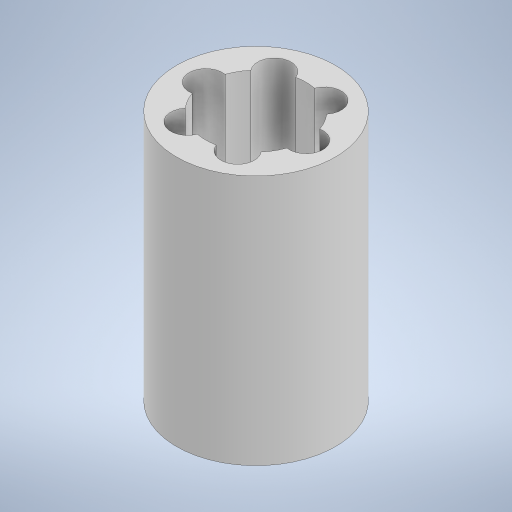
# Autodesk Inventor part: Bearing
Saved by Autodesk Inventor 2023 (Build 270158000, 158)
## iProperties
Created: 2023-04-11
Part Number: Bearing
Material: Generic
Document SubType Name: Modeling
Designer: Nathann
Density: 1 g/cm^3
Appearance: Default
Author: Nathann
Autodesk Inventor part; units mm, degrees
ref_plane "YZ Plane" through (0, 0, 0) normal (1, 0, 0) x (0, 1, 0)
ref_plane "XZ Plane" through (0, 0, 0) normal (0, 1, 0) x (-1, 0, 0)
ref_plane "XY Plane" through (0, 0, 0) normal (0, 0, 1) x (1, 0, 0)
sketch "Sketch1" plane through (0, 0, 0) normal (0, 1, 0) x (-1, 0, 0)
  circle A0 centre (0, 0) radius 6
  circle A1 centre (0, 0) radius 9.5
  circle A2 centre (6, 0) radius 2
  circle A3 centre (3, 5.1962) radius 2
  circle A4 centre (-3, 5.1962) radius 2
  circle A5 centre (-6, 0) radius 2
  circle A6 centre (-3, -5.1962) radius 2
  circle A7 centre (3, -5.1962) radius 2
  point P0 (5.6667, -1.972)
  point P1 (5.6667, 1.972)
  point P2 (4.5412, -3.9215)
  point P3 (1.1255, -5.8935)
  point P4 (-1.1255, -5.8935)
  point P5 (-4.5412, -3.9215)
  point P6 (-5.6667, -1.972)
  point P7 (-5.6667, 1.972)
  point P8 (-4.5412, 3.9215)
  point P9 (-1.1255, 5.8935)
  point P10 (1.1255, 5.8935)
  point P11 (4.5412, 3.9215)
  dimension "d1" = 12
  dimension "d0" = 19
  dimension "d2" = 4
  dimension "d7" = 360
  dimension "d9" = 6
  dimension "d10" = 5.1962
  dimension "d11" = 3
  dimension "d12" = 3
  constraints: 7 centre point, 2 coincident, 16 other
  measures "d0" diameter of A1
  measures "d2" diameter of A2
  measures "d9" distance of point (0, 0) A2.centre
  measures "d10" vertical distance of A7.centre point (0, 0)
  measures "d11" horizontal distance of A7.centre point (0, 0)
  measures "d12" horizontal distance of A6.centre point (0, 0)
extrude "Extrusion1" add sketch "Sketch1" along normal blind 30
body "Solid1"
